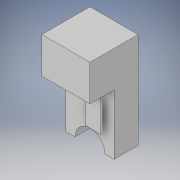
# Autodesk Inventor part: graber base
Saved by Autodesk Inventor 2019 (Build 230136000, 136)
## iProperties
Created: 2020-10-22
Part Number: graber base
Material: Generic
Document SubType Name: Modeling
Designer: User
Density: 1 g/cm^3
Appearance: Default
Author: User
Autodesk Inventor part; units mm, degrees
ref_plane "YZ Plane" through (0, 0, 0) normal (1, 0, 0) x (0, 1, 0)
ref_plane "XZ Plane" through (0, 0, 0) normal (0, 1, 0) x (-1, 0, 0)
ref_plane "XY Plane" through (0, 0, 0) normal (0, 0, 1) x (1, 0, 0)
sketch "Sketch4" plane through (0, 0, 0) normal (1, 0, 0) x (0, 1, 0)
  line L0 (0, 0) -> (-101.6, 0)
  line L1 (-101.6, 0) -> (-101.6, -50.8)
  line L2 (-101.6, -50.8) -> (0, -50.8)
  line L3 (0, -50.8) -> (0, 0)
  dimension "d6" = 101.6
  dimension "d7" = 50.8
  constraints: 8 end point, 2 parallel, 1 horizontal, 1 perpendicular
  measures "d6" distance of L2.end L1.end
  measures "d7" distance of L1.end L0.end
extrude "Extrusion3" add sketch "Sketch4" along normal blind 50.8
sketch "Sketch5" plane through (0, -101.6, 0) normal (0, 0, 1) x (1, 0, 0)
  line L0 (0, 0) -> (50.8, 0) projected
  arc A0 (41.275, 0) -> (9.525, 0) centre (25.4, 0) ccw
  line L1 (0, 101.6) -> (0, 0) projected
  dimension "d10" = 15.875
  dimension "d11" = 31.75
  dimension "d12" = 50.8
  dimension "d13" = 9.525
  constraints: 2 point on circle, 2 point on line, 1 centre point
  measures "d10" radius of A0
  measures "d11" distance of A0.start A0.end
  measures "d12" distance of L0.start L0.end
  measures "d13" distance from line of L1 A0.end
extrude "Extrusion4" cut sketch "Sketch5" against normal through all
sketch "Sketch6" plane through (0, -101.6, -50.8) normal (0, -1, 0) x (1, 0, 0)
  line L0 (0, 50.8) -> (9.525, 50.8) projected
  line L1 (50.8, 50.8) -> (50.8, 0) projected
  line L2 (0, 50.8) -> (50.8, 50.8)
  line L3 (50.8, 50.8) -> (50.8, 25.4)
  line L4 (50.8, 25.4) -> (0, 25.4)
  line L5 (0, 25.4) -> (0, 50.8)
  constraints: 8 end point, 2 parallel, 1 horizontal, 1 midpoint, 1 perpendicular
extrude "Extrusion5" cut sketch "Sketch6" against normal blind 63.5
sketch "Sketch7" plane through (0, -38.1, -50.8) normal (0, -1, 0) x (1, 0, 0)
  line L0 (46.6725, 33.9725) -> (29.5275, 33.9725) construction
  line L1 (45.72, 34.925) -> (30.48, 34.925)
  line L2 (30.48, 33.02) -> (45.72, 33.02)
  arc A0 (45.72, 33.02) -> (45.72, 34.925) centre (45.72, 33.9725) ccw
  arc A1 (30.48, 34.925) -> (30.48, 33.02) centre (30.48, 33.9725) ccw
  line L3 (0, 50.8) -> (50.8, 50.8) projected
  line L4 (50.8, 50.8) -> (50.8, 25.4) projected
  line L5 (41.275, 25.4) -> (9.525, 25.4) projected
  point P0 (38.1, 33.9725)
  dimension "d18" = 17.145
  dimension "d19" = 1.905
  dimension "d20" = 50.8
  dimension "d21" = 4.1275
  dimension "d22" = 7.62
  constraints: 8 end point, 6 point on circle, 4 tangent, 2 centre point, 2 parallel, 2 point on line, 1 midpoint
  measures "d18" distance of L0.start L0.end
  measures "d19" diameter of A1
  measures "d20" distance of L3.start L3.end
  measures "d21" distance from line of L4 L0.start
  measures "d22" distance between parallel lines of L5 L2
extrude "Extrusion6" add sketch "Sketch7" along normal blind 38.1
equation "\"d13\" = -0.5 * d11 + 0.5 * d12"
body "Solid2"
